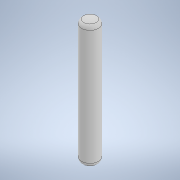
# Autodesk Inventor part: Volume Test Part
Saved by Autodesk Inventor 2021 (Build 250183000, 183)
## iProperties
Created: 2021-09-28
Part Number: Volume Test Part
Material: Generic
Document SubType Name: Modeling
Designer: Alex Clay
Mass: 272379 g
Surface Area: 39843.8 cm^2
Volume: 272379 cm^3
Density: 1 g/cm^3
Appearance: Default
Author: Alex Clay
Autodesk Inventor part; units mm, degrees
ref_plane "YZ Plane" through (0, 0, 0) normal (1, 0, 0) x (0, 1, 0)
ref_plane "XZ Plane" through (0, 0, 0) normal (0, 1, 0) x (-1, 0, 0)
ref_plane "XY Plane" through (0, 0, 0) normal (0, 0, 1) x (1, 0, 0)
sketch "Sketch3" plane through (0, 0, 0) normal (0, 0, 1) x (1, 0, 0)
  line L0 (0, 0) -> (139.7, 0)
  line L1 (139.7, 0) -> (139.7, 952.5)
  arc A0 (139.7, 952.5) -> (101.7568, 1016.9811) centre (65.9384, 952.5) ccw
  arc A1 (101.7568, 1016.9811) -> (0, 1043.3461) centre (0, 833.7961) ccw
  line L2 (0, 1043.3461) -> (0, 0)
  dimension "d3" = 139.7
  dimension "d4" = 952.5
  dimension "d5" = 73.7616
  dimension "d6" = 209.55
  constraints: 6 end point, 5 point on circle, 2 centre point, 2 tangent, 1 horizontal, 1 perpendicular, 1 point on line, 1 vertical
  measures "d3" distance of L0.start L0.end
  measures "d4" distance of L0.end L1.end
  measures "d5" radius of A0
  measures "d6" radius of A1
revolve "Revolution1" add sketch "Sketch3" angle 360 about axis through (0, 1043.3461, 0) along (0, -1, 0)
mirror "Mirror1" about plane through (0, 0, 0) normal (0, -1, 0)
equation "\"d4\" = 0.5 * Height"
equation "\"d5\" = 0.528 * d3"
equation "\"d6\" = 1.5 * d3"
equation "\"Diameter\" = 304.8"
equation "\"Height\" = 1905"
body "Solid2"
